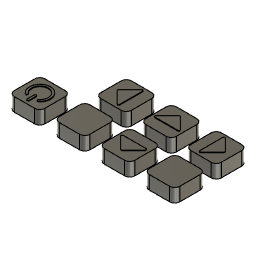
Buttons (Autodesk Fusion 360 design; units mm, degrees)
Autodesk Fusion 360 part; units mm, degrees
sketch "Sketch1" plane through (0, 0, 0) normal (0, 0, 1) x (1, 0, 0)
  line L0 (-42.0668, -28.6036) -> (-22.5668, -28.6036)
  line L1 (-17.5668, -33.6036) -> (-17.5668, -53.1036)
  line L2 (-22.5668, -58.1036) -> (-42.0668, -58.1036)
  line L3 (-47.0668, -53.1036) -> (-47.0668, -33.6036)
  arc A0 (-42.0668, -28.6036) -> (-47.0668, -33.6036) centre (-42.0668, -33.6036) ccw
  arc A1 (-17.5668, -33.6036) -> (-22.5668, -28.6036) centre (-22.5668, -33.6036) ccw
  arc A2 (-22.5668, -58.1036) -> (-17.5668, -53.1036) centre (-22.5668, -53.1036) ccw
  arc A3 (-47.0668, -53.1036) -> (-42.0668, -58.1036) centre (-42.0668, -53.1036) ccw
  arc A4 (20.7666, -58.1036) -> (25.7666, -53.1036) centre (20.7666, -53.1036) ccw
  arc A5 (1.2666, -28.6036) -> (-3.7334, -33.6036) centre (1.2666, -33.6036) ccw
  line L4 (-3.7334, -53.1036) -> (-3.7334, -33.6036)
  line L5 (20.7666, -58.1036) -> (1.2666, -58.1036)
  arc A6 (25.7666, -33.6036) -> (20.7666, -28.6036) centre (20.7666, -33.6036) ccw
  arc A7 (-3.7334, -53.1036) -> (1.2666, -58.1036) centre (1.2666, -53.1036) ccw
  line L6 (1.2666, -28.6036) -> (20.7666, -28.6036)
  line L7 (25.7666, -33.6036) -> (25.7666, -53.1036)
  arc A8 (64.0999, -58.1036) -> (69.0999, -53.1036) centre (64.0999, -53.1036) ccw
  arc A9 (44.5999, -28.6036) -> (39.5999, -33.6036) centre (44.5999, -33.6036) ccw
  line L8 (39.5999, -53.1036) -> (39.5999, -33.6036)
  line L9 (64.0999, -58.1036) -> (44.5999, -58.1036)
  arc A10 (69.0999, -33.6036) -> (64.0999, -28.6036) centre (64.0999, -33.6036) ccw
  arc A11 (39.5999, -53.1036) -> (44.5999, -58.1036) centre (44.5999, -53.1036) ccw
  line L10 (44.5999, -28.6036) -> (64.0999, -28.6036)
  line L11 (69.0999, -33.6036) -> (69.0999, -53.1036)
  arc A12 (107.4332, -58.1036) -> (112.4332, -53.1036) centre (107.4332, -53.1036) ccw
  arc A13 (87.9332, -28.6036) -> (82.9332, -33.6036) centre (87.9332, -33.6036) ccw
  line L12 (82.9332, -53.1036) -> (82.9332, -33.6036)
  line L13 (107.4332, -58.1036) -> (87.9332, -58.1036)
  arc A14 (112.4332, -33.6036) -> (107.4332, -28.6036) centre (107.4332, -33.6036) ccw
  arc A15 (82.9332, -53.1036) -> (87.9332, -58.1036) centre (87.9332, -53.1036) ccw
  line L14 (87.9332, -28.6036) -> (107.4332, -28.6036)
  line L15 (112.4332, -33.6036) -> (112.4332, -53.1036)
  arc A16 (20.7666, -18.1036) -> (25.7666, -13.1036) centre (20.7666, -13.1036) ccw
  arc A17 (1.2666, 11.3964) -> (-3.7334, 6.3964) centre (1.2666, 6.3964) ccw
  line L16 (-3.7334, -13.1036) -> (-3.7334, 6.3964)
  line L17 (20.7666, -18.1036) -> (1.2666, -18.1036)
  arc A18 (25.7666, 6.3964) -> (20.7666, 11.3964) centre (20.7666, 6.3964) ccw
  arc A19 (-3.7334, -13.1036) -> (1.2666, -18.1036) centre (1.2666, -13.1036) ccw
  line L18 (1.2666, 11.3964) -> (20.7666, 11.3964)
  line L19 (25.7666, 6.3964) -> (25.7666, -13.1036)
  arc A20 (64.0999, -18.1036) -> (69.0999, -13.1036) centre (64.0999, -13.1036) ccw
  arc A21 (44.5999, 11.3964) -> (39.5999, 6.3964) centre (44.5999, 6.3964) ccw
  line L20 (39.5999, -13.1036) -> (39.5999, 6.3964)
  line L21 (64.0999, -18.1036) -> (44.5999, -18.1036)
  arc A22 (69.0999, 6.3964) -> (64.0999, 11.3964) centre (64.0999, 6.3964) ccw
  arc A23 (39.5999, -13.1036) -> (44.5999, -18.1036) centre (44.5999, -13.1036) ccw
  line L22 (44.5999, 11.3964) -> (64.0999, 11.3964)
  line L23 (69.0999, 6.3964) -> (69.0999, -13.1036)
  arc A24 (107.4332, -18.1036) -> (112.4332, -13.1036) centre (107.4332, -13.1036) ccw
  arc A25 (87.9332, 11.3964) -> (82.9332, 6.3964) centre (87.9332, 6.3964) ccw
  line L24 (82.9332, -13.1036) -> (82.9332, 6.3964)
  line L25 (107.4332, -18.1036) -> (87.9332, -18.1036)
  arc A26 (112.4332, 6.3964) -> (107.4332, 11.3964) centre (107.4332, 6.3964) ccw
  arc A27 (82.9332, -13.1036) -> (87.9332, -18.1036) centre (87.9332, -13.1036) ccw
  line L26 (87.9332, 11.3964) -> (107.4332, 11.3964)
  line L27 (112.4332, 6.3964) -> (112.4332, -13.1036)
  line L28 (54.3499, -58.1036) -> (54.3499, -52.1036)
  line L29 (55.057, -51.3965) -> (66.1428, -40.3107)
  line L30 (65.4357, -38.6036) -> (43.2641, -38.6036)
  line L31 (42.557, -40.3107) -> (53.6428, -51.3965)
  arc A28 (66.1428, -40.3107) -> (65.4357, -38.6036) centre (65.4357, -39.6036) ccw
  arc A29 (43.2641, -38.6036) -> (42.557, -40.3107) centre (43.2641, -39.6036) ccw
  arc A30 (53.6428, -51.3965) -> (55.057, -51.3965) centre (54.3499, -50.6894) ccw
  line L32 (54.3499, 11.3964) -> (54.3499, 5.3964)
  line L33 (53.6428, 4.6893) -> (42.557, -6.3965)
  line L34 (43.2641, -8.1036) -> (65.4357, -8.1036)
  line L35 (66.1428, -6.3965) -> (55.057, 4.6893)
  arc A31 (65.4357, -8.1036) -> (66.1428, -6.3965) centre (65.4357, -7.1036) ccw
  arc A32 (42.557, -6.3965) -> (43.2641, -8.1036) centre (43.2641, -7.1036) ccw
  arc A33 (55.057, 4.6893) -> (53.6428, 4.6893) centre (54.3499, 3.9821) ccw
  line L36 (112.4332, -3.3536) -> (106.4332, -3.3536)
  line L37 (-3.7334, -3.3536) -> (2.2666, -3.3536)
  line L38 (105.7261, -4.0607) -> (94.6403, -15.1465)
  line L39 (92.9332, -14.4394) -> (92.9332, 7.7321)
  line L40 (94.6403, 8.4393) -> (105.7261, -2.6465)
  line L41 (2.9737, -4.0607) -> (14.0594, -15.1465)
  line L42 (15.7666, -14.4394) -> (15.7666, 7.7321)
  line L43 (14.0594, 8.4393) -> (2.9737, -2.6465)
  arc A34 (92.9332, -14.4394) -> (94.6403, -15.1465) centre (93.9332, -14.4394) ccw
  arc A35 (94.6403, 8.4393) -> (92.9332, 7.7321) centre (93.9332, 7.7321) ccw
  arc A36 (105.7261, -4.0607) -> (105.7261, -2.6465) centre (105.019, -3.3536) ccw
  arc A37 (14.0594, -15.1465) -> (15.7666, -14.4394) centre (14.7666, -14.4394) ccw
  arc A38 (15.7666, 7.7321) -> (14.0594, 8.4393) centre (14.7666, 7.7321) ccw
  arc A39 (2.9737, -2.6465) -> (2.9737, -4.0607) centre (3.6808, -3.3536) ccw
  arc A40 (-26.0406, -50.8888) -> (-38.593, -50.8888) centre (-32.3168, -43.1036) ccw
  arc A41 (-27.2958, -49.3318) -> (-37.3378, -49.3318) centre (-32.3168, -43.1036) ccw
  arc A42 (-27.2958, -49.3318) -> (-26.0406, -50.8888) centre (-26.6682, -50.1103) ccw
  arc A43 (-38.593, -50.8888) -> (-37.3378, -49.3318) centre (-37.9654, -50.1103) ccw
  line L44 (-31.3168, -54.6036) -> (-31.3168, -47.6036)
  arc A44 (-31.3168, -47.6036) -> (-33.3168, -47.6036) centre (-32.3168, -47.6036) ccw
  line L45 (-33.3168, -47.6036) -> (-33.3168, -54.6036)
  arc A45 (-33.3168, -54.6036) -> (-31.3168, -54.6036) centre (-32.3168, -54.6036) ccw
  line L46 (-32.3168, -54.6036) -> (-32.3168, -47.6036) construction
  point P0 (-47.0668, -28.6036)
  point P1 (-17.5668, -28.6036)
  point P2 (-47.0668, -58.1036)
  point P3 (-3.7334, -58.1036)
  point P4 (25.7666, -28.6036)
  point P5 (-3.7334, -28.6036)
  point P6 (39.5999, -58.1036)
  point P7 (69.0999, -28.6036)
  point P8 (39.5999, -28.6036)
  point P9 (82.9332, -58.1036)
  point P10 (112.4332, -28.6036)
  point P11 (82.9332, -28.6036)
  point P12 (-3.7334, -18.1036)
  point P13 (25.7666, 11.3964)
  point P14 (-3.7334, 11.3964)
  point P15 (39.5999, -18.1036)
  point P16 (69.0999, 11.3964)
  point P17 (39.5999, 11.3964)
  point P18 (82.9332, -18.1036)
  point P19 (112.4332, 11.3964)
  point P20 (82.9332, 11.3964)
  dimension "d15" = 29.5
  dimension "d16" = 29.5
  dimension "d17" = 5
  dimension "d18" = 5
  dimension "d21" = 130
  dimension "d22" = 40
  dimension "d23" = 6
  dimension "d24" = 45
  dimension "d25" = 45
  dimension "d26" = 10
  dimension "d27" = 1
  dimension "d28" = 1
  dimension "d29" = 1
  dimension "d30" = 6
  dimension "d31" = 45
  dimension "d32" = 45
  dimension "d33" = 10
  dimension "d34" = 1
  dimension "d35" = 1
  dimension "d36" = 1
  dimension "d37" = 6
  dimension "d38" = 6
  dimension "d39" = 45
  dimension "d40" = 45
  dimension "d41" = 45
  dimension "d42" = 45
  dimension "d43" = 10
  dimension "d44" = 10
  dimension "d45" = 1
  dimension "d46" = 1
  dimension "d47" = 1
  dimension "d48" = 1
  dimension "d49" = 1
  dimension "d50" = 1
  dimension "d51" = 20
  dimension "d52" = 16
  dimension "d54" = 2
  dimension "d55" = 7
  dimension "d56" = 3.5
  dimension "d61" = 14.75
  dimension "d62" = 14.75
  constraint horizontal L0
  constraint vertical L1
  constraint horizontal L2
  constraint vertical L3
  constraint coincident P0 L0
  constraint coincident P0 L3
  constraint tangent L0 A0
  constraint tangent L3 A0
  constraint coincident P1 L0
  constraint coincident P1 L1
  constraint tangent L0 A1
  constraint tangent L1 A1
  constraint equal A0 A1
  constraint tangent L1 A2
  constraint tangent L2 A2
  constraint equal A0 A2
  constraint coincident P2 L2
  constraint coincident P2 L3
  constraint tangent L2 A3
  constraint tangent L3 A3
  constraint midpoint L9 L28.start
  constraint perpendicular L9 L28
  constraint perpendicular L28 L30
  constraint tangent L29 A28
  constraint tangent L30 A28
  constraint tangent L30 A29
  constraint tangent L31 A29
  constraint coincident L28.end L31
  constraint coincident L28.end L29
  constraint tangent L31 A30
  constraint tangent L29 A30
  constraint midpoint L22 L32.start
  constraint perpendicular L22 L32
  constraint perpendicular L32 L34
  constraint tangent L34 A31
  constraint tangent L35 A31
  constraint tangent L33 A32
  constraint tangent L34 A32
  constraint coincident L32.end L33
  constraint coincident L32.end L35
  constraint tangent L33 A33
  constraint tangent L35 A33
  constraint midpoint L27 L36.start
  constraint perpendicular L27 L36
  constraint midpoint L16 L37.start
  constraint perpendicular L16 L37
  constraint perpendicular L36 L39
  constraint vertical L42
  constraint tangent L38 A34
  constraint tangent L39 A34
  constraint tangent L39 A35
  constraint tangent L40 A35
  constraint coincident L36.end L40
  constraint coincident L36.end L38
  constraint tangent L40 A36
  constraint tangent L38 A36
  constraint tangent L41 A37
  constraint tangent L42 A37
  constraint tangent L42 A38
  constraint tangent L43 A38
  constraint coincident L37.end L41
  constraint coincident L37.end L43
  constraint tangent L41 A39
  constraint tangent L43 A39
  constraint concentric A40 A41
  constraint tangent A40 A42
  constraint tangent A41 A42
  constraint tangent A40 A43
  constraint tangent A41 A43
  constraint horizontal A42.centre A43.centre
  constraint tangent L44 A44
  constraint tangent A44 L45
  constraint parallel L44 L45
  constraint tangent L45 A45
  constraint tangent L44 A45
  constraint perpendicular L2 L46
  measures "d15" distance of P0 P1
  measures "d16" distance of P0 P2
  measures "d17" radius of A0
  measures "d18" radius of A3
  measures "d23" distance of L28.start L28.end
  measures "d24" angle of L29 L30
  measures "d25" angle of L30 L31
  measures "d26" distance of L10 L30
  measures "d27" radius of A28
  measures "d28" radius of A29
  measures "d29" radius of A30
  measures "d30" distance of L32.start L32.end
  measures "d31" angle of L34 L35
  measures "d32" angle of L33 L34
  measures "d33" distance of L21 L34
  measures "d34" radius of A31
  measures "d35" radius of A32
  measures "d36" radius of A33
  measures "d37" distance of L36.start L36.end
  measures "d38" distance of L37.start L37.end
  measures "d39" angle of L41 L42
  measures "d40" angle of L42 L43
  measures "d41" angle of L38 L39
  measures "d42" angle of L39 L40
  measures "d43" distance of L24 L39
  measures "d44" distance of L19 L42
  measures "d45" radius of A34
  measures "d46" radius of A35
  measures "d47" radius of A36
  measures "d48" radius of A37
  measures "d49" radius of A38
  measures "d50" radius of A39
  measures "d51" diameter of A40
  measures "d52" diameter of A41
  measures "d54" diameter of A44
  measures "d55" distance of A45.centre A44.centre
  measures "d56" distance of L2 A45.centre
  measures "d61" distance of L3 A40.centre
  measures "d62" distance of L3 L46
extrude "Extrude1" add sketch "Sketch1" along normal blind 0.6 contours L29 L30 L31 A28 A29 A30 | L33 L34 L35 A31 A32 A33 | L38 L39 L40 A34 A35 A36 | L41 L42 L43 A37 A38 A39 | A40 A41 A42 A43 | L44 A44 L45 A45 makes body 1 at (54.1142, -42.8679, 0) makes body 2 at (11.5023, -3.1179, 0) makes body 3 at (-23.2784, -45.3338, 0) makes body 4 at (97.1975, -3.1179, 0) makes body 5 at (54.5856, -3.8393, 0) makes body 6 at (-32.6501, -49.937, 0)
extrude "Extrude2" add sketch "Sketch1" against normal blind 13 separate body contours L0 L1 L2 L3 A0 A1 A2 A3 | A4 A5 L4 L5 A6 A7 L6 L7 | A8 A9 L8 L9 A10 A11 L10 L11 | A12 A13 L12 L13 A14 A15 L14 L15 | A16 A17 L16 L17 A18 A19 L18 L19 | A20 A21 L20 L21 A22 A23 L22 L23 | A24 A25 L24 L25 A26 A27 L26 L27 | L29 L30 L31 A28 A29 A30 | L33 L34 L35 A31 A32 A33 | L38 L39 L40 A34 A35 A36 | L41 L42 L43 A37 A38 A39 | A40 A41 A42 A43 | L44 A44 L45 A45 makes body 7 at (57.5999, -44.937, 0) makes body 8 at (14.2666, -4.937, 0) makes body 9 at (-29.0668, -48.2703, 0) makes body 10 at (51.0999, 1.563, 0) makes body 11 at (102.5999, -0.1036, 0) makes body 12 at (15.9332, -46.6036, 0) makes body 13 at (100.9332, -38.437, 0)
